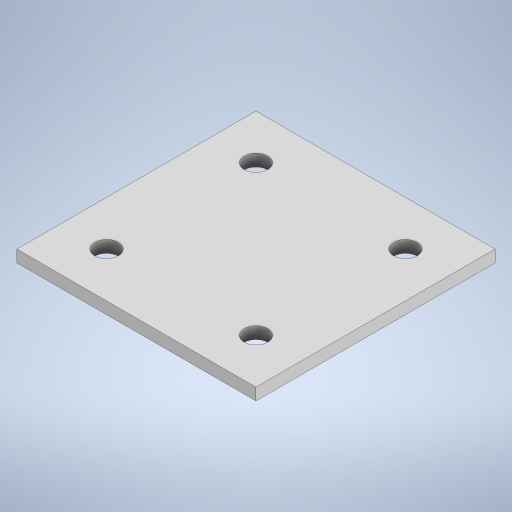
# Autodesk Inventor part: l channel guide
Saved by Autodesk Inventor 2024 (Build 280153000, 153)
## iProperties
Created: 2024-06-21
Part Number: l channel guide
Material: Generic
Document SubType Name: Modeling
Designer: ony
Density: 1 g/cm^3
Appearance: Default
Author: ony
Autodesk Inventor part; units mm, degrees
ref_plane "YZ Plane" through (0, 0, 0) normal (1, 0, 0) x (0, 1, 0)
ref_plane "XZ Plane" through (0, 0, 0) normal (0, 1, 0) x (-1, 0, 0)
ref_plane "XY Plane" through (0, 0, 0) normal (0, 0, 1) x (1, 0, 0)
sketch "Sketch1" plane through (0, 0, 0) normal (0, 1, 0) x (-1, 0, 0)
  line L0 (-25.4, -25.4) -> (25.4, -25.4)
  line L1 (25.4, -25.4) -> (25.4, 25.4)
  line L2 (25.4, 25.4) -> (-25.4, 25.4)
  line L3 (-25.4, 25.4) -> (-25.4, -25.4)
  line L4 (-25.4, -25.4) -> (25.4, 25.4) construction
  line L5 (25.4, -25.4) -> (-25.4, 25.4) construction
  line L6 (-15.875, 15.875) -> (15.875, 15.875)
  line L7 (15.875, 15.875) -> (15.875, -15.875)
  line L8 (15.875, -15.875) -> (-15.875, -15.875)
  line L9 (-15.875, -15.875) -> (-15.875, 15.875)
  line L10 (-15.875, 15.875) -> (15.875, -15.875) construction
  line L11 (15.875, 15.875) -> (-15.875, -15.875) construction
  circle A0 centre (15.875, 15.875) radius 2.5
  circle A1 centre (15.875, -15.875) radius 2.5
  circle A2 centre (-15.875, -15.875) radius 2.5
  circle A3 centre (-15.875, 15.875) radius 2.5
  point P0 (0, 0)
  dimension "d0" = 50.8
  dimension "d1" = 50.8
  dimension "d2" = 31.75
  dimension "d3" = 31.75
  dimension "d4" = 5
  dimension "d5" = 5
  dimension "d6" = 5
  dimension "d7" = 5
  constraints: 24 end point, 4 centre point, 4 midpoint, 4 parallel, 3 coincident, 2 horizontal, 2 perpendicular, 1 point on line
  measures "d0" distance of L2.end L1.end
  measures "d1" distance of L1.end L0.end
  measures "d2" distance of L7.end L8.end
  measures "d3" distance of L6.end L7.end
  measures "d4" diameter of A0
  measures "d5" diameter of A1
  measures "d6" diameter of A2
  measures "d7" diameter of A3
extrude "Extrusion1" add sketch "Sketch1" along normal blind 2.54 contours L3 L2 L1 L0 | L6 A0 L7 A1 L8 A2 L9 A3
body "Solid1"
